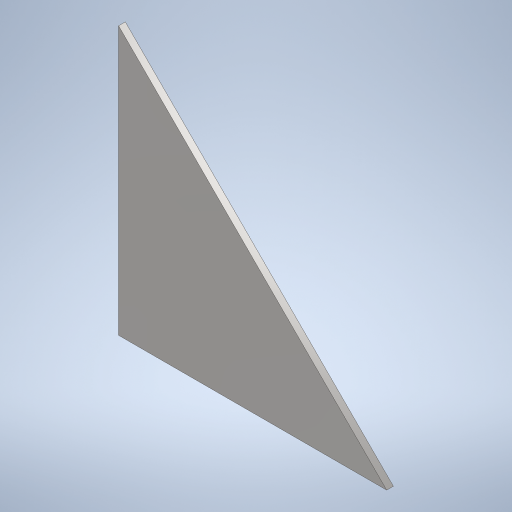
# Autodesk Inventor part: kat
Saved by Autodesk Inventor 2023 (Build 270158000, 158)
## iProperties
Created: 2023-06-13
Part Number: kat
Material: Stal, miękka
Document SubType Name: Modeling
Designer: MateuszWawrzyniak
Density: 7.85 g/cm^3
Appearance: Częściowo polerowany
Author: MateuszWawrzyniak
Autodesk Inventor part; units mm, degrees
ref_plane "YZ Plane" through (0, 0, 0) normal (1, 0, 0) x (0, 1, 0)
ref_plane "XZ Plane" through (0, 0, 0) normal (0, 1, 0) x (-1, 0, 0)
ref_plane "XY Plane" through (0, 0, 0) normal (0, 0, 1) x (1, 0, 0)
sketch "Szkic1" plane through (0, 0, 0) normal (0, 0, 1) x (1, 0, 0)
  line L0 (0, 0) -> (200, 0)
  line L1 (0, 0) -> (0, 200)
  line L2 (0, 200) -> (200, 0)
  dimension "d0" = 200
  dimension "d1" = 200
  constraints: 6 end point, 1 horizontal, 1 vertical
  measures "d0" distance of L0.start L0.end
  measures "d1" distance of L0.start L1.end
extrude "Wyciągnięcie proste1" add sketch "Szkic1" along normal blind 5
